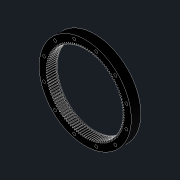
# Autodesk Inventor part: unit-ring_gear
Saved by Autodesk Inventor 2022 (Build 260153000, 153)
## iProperties
Created: 2021-07-12
Part Number: unit-ring_gear
Material: ABS プラスチック
Document SubType Name: Modeling
Designer: yuta0
Density: 1.06 g/cm^3
Appearance: 滑らか - 黒
Mass: 40.8022 g
Surface Area: 244.347 cm^2
Volume: 38.4926 cm^3
購入先: 印刷
在庫数: 0.0
Author: yuta0
Autodesk Inventor part; units mm, degrees
ref_plane "YZ Plane" through (0, 0, 0) normal (1, 0, 0) x (0, 1, 0)
ref_plane "XZ Plane" through (0, 0, 0) normal (0, 1, 0) x (-1, 0, 0)
ref_plane "XY Plane" through (0, 0, 0) normal (0, 0, 1) x (1, 0, 0)
sketch "スケッチ1" plane through (0, 0, 0) normal (0, 0, 1) x (1, 0, 0)
  circle A0 centre (0, 0) radius 67.5
  arc A1 (3.6193, -57.2712) -> (4.2488, -54.9715) centre (-9.8202, -52.3566) ccw
  arc A2 (2.8158, -57.3163) -> (3.6193, -57.2712) centre (0, 0) ccw
  arc A3 (1.9328, -55.1015) -> (2.8158, -57.3163) centre (15.6206, -50.9279) ccw
  arc A4 (1.1598, -55.1232) -> (1.9328, -55.1015) centre (0, 0) ccw
  arc A5 (0.4024, -57.384) -> (1.1598, -55.1232) centre (-12.7405, -51.7236) ccw
  arc A6 (-0.4024, -57.384) -> (0.4024, -57.384) centre (0, 0) ccw
  arc A7 (-1.1598, -55.1232) -> (-0.4024, -57.384) centre (12.7405, -51.7236) ccw
  arc A8 (-1.9328, -55.1015) -> (-1.1598, -55.1232) centre (0, 0) ccw
  arc A9 (-2.8158, -57.3163) -> (-1.9328, -55.1015) centre (-15.6206, -50.9279) ccw
  arc A10 (-3.6193, -57.2712) -> (-2.8158, -57.3163) centre (0, 0) ccw
  arc A11 (-4.2488, -54.9715) -> (-3.6193, -57.2712) centre (9.8202, -52.3566) ccw
  arc A12 (-5.0193, -54.9065) -> (-4.2488, -54.9715) centre (0, 0) ccw
  arc A13 (-6.0251, -57.0682) -> (-5.0193, -54.9065) centre (-18.4516, -49.9719) ccw
  arc A14 (-6.8249, -56.9781) -> (-6.0251, -57.0682) centre (0, 0) ccw
  arc A15 (-7.3244, -54.6468) -> (-6.8249, -56.9781) centre (6.8691, -52.8248) ccw
  arc A16 (-8.09, -54.5387) -> (-7.3244, -54.6468) centre (0, 0) ccw
  arc A17 (-9.2155, -56.6406) -> (-8.09, -54.5387) centre (-21.2245, -48.8587) ccw
  arc A18 (-10.0089, -56.5058) -> (-9.2155, -56.6406) centre (0, 0) ccw
  arc A19 (-10.3769, -54.1501) -> (-10.0089, -56.5058) centre (3.8964, -53.1269) ccw
  arc A20 (-11.1353, -53.9992) -> (-10.3769, -54.1501) centre (0, 0) ccw
  arc A21 (-12.3768, -56.0348) -> (-11.1353, -53.9992) centre (-23.9306, -47.5918) ccw
  arc A22 (-13.1615, -55.8557) -> (-12.3768, -56.0348) centre (0, 0) ccw
  arc A23 (-13.3968, -53.4831) -> (-13.1615, -55.8557) centre (0.9114, -53.2618) ccw
  arc A24 (-14.1456, -53.2899) -> (-13.3968, -53.4831) centre (0, 0) ccw
  arc A25 (-15.4992, -55.2527) -> (-14.1456, -53.2899) centre (-26.5615, -46.1751) ccw
  arc A26 (-16.2726, -55.0299) -> (-15.4992, -55.2527) centre (0, 0) ccw
  arc A27 (-16.3746, -52.6478) -> (-16.2726, -55.0299) centre (-2.0764, -53.2291) ccw
  arc A28 (-17.1113, -52.4129) -> (-16.3746, -52.6478) centre (0, 0) ccw
  arc A29 (-18.5729, -54.2967) -> (-17.1113, -52.4129) centre (-29.1087, -44.6131) ccw
  arc A30 (-19.3326, -54.0309) -> (-18.5729, -54.2967) centre (0, 0) ccw
  arc A31 (-19.3008, -51.6468) -> (-19.3326, -54.0309) centre (-5.0577, -53.0289) ccw
  arc A32 (-20.0232, -51.3711) -> (-19.3008, -51.6468) centre (0, 0) ccw
  arc A33 (-21.5881, -53.1699) -> (-20.0232, -51.3711) centre (-31.5644, -42.9108) ccw
  arc A34 (-22.3317, -52.8619) -> (-21.5881, -53.1699) centre (0, 0) ccw
  arc A35 (-22.1663, -50.4834) -> (-22.3317, -52.8619) centre (-8.0231, -52.6619) ccw
  arc A36 (-22.8721, -50.1675) -> (-22.1663, -50.4834) centre (0, 0) ccw
  arc A37 (-24.5354, -51.8758) -> (-22.8721, -50.1675) centre (-33.9208, -41.0735) ccw
  arc A38 (-25.2605, -51.5266) -> (-24.5354, -51.8758) centre (0, 0) ccw
  arc A39 (-24.962, -49.1611) -> (-25.2605, -51.5266) centre (-10.9633, -52.1292) ccw
  arc A40 (-25.649, -48.8062) -> (-24.962, -49.1611) centre (0, 0) ccw
  arc A41 (-27.4055, -50.4185) -> (-25.649, -48.8062) centre (-36.1704, -39.1069) ccw
  arc A42 (-28.1099, -50.0292) -> (-27.4055, -50.4185) centre (0, 0) ccw
  arc A43 (-27.6792, -47.6841) -> (-28.1099, -50.0292) centre (-13.8689, -51.4325) ccw
  arc A44 (-28.3453, -47.2912) -> (-27.6792, -47.6841) centre (0, 0) ccw
  arc A45 (-30.1894, -48.8025) -> (-28.3453, -47.2912) centre (-38.3063, -37.0173) ccw
  arc A46 (-30.8709, -48.3743) -> (-30.1894, -48.8025) centre (0, 0) ccw
  arc A47 (-30.3094, -46.0571) -> (-30.8709, -48.3743) centre (-16.731, -50.574) ccw
  arc A48 (-30.9523, -45.6275) -> (-30.3094, -46.0571) centre (0, 0) ccw
  arc A49 (-32.8783, -47.033) -> (-30.9523, -45.6275) centre (-40.3216, -34.8112) ccw
  arc A50 (-33.5347, -46.5673) -> (-32.8783, -47.033) centre (0, 0) ccw
  arc A51 (-32.8441, -44.2852) -> (-33.5347, -46.5673) centre (-19.5403, -49.5563) ccw
  arc A52 (-33.462, -43.8202) -> (-32.8441, -44.2852) centre (0, 0) ccw
  arc A53 (-35.4637, -45.1155) -> (-33.462, -43.8202) centre (-42.21, -32.4956) ccw
  arc A54 (-36.093, -44.6137) -> (-35.4637, -45.1155) centre (0, 0) ccw
  arc A55 (-35.2755, -42.3739) -> (-36.093, -44.6137) centre (-22.2882, -48.3827) ccw
  arc A56 (-35.8664, -41.875) -> (-35.2755, -42.3739) centre (0, 0) ccw
  arc A57 (-37.9376, -43.0561) -> (-35.8664, -41.875) centre (-43.9657, -30.0777) ccw
  arc A58 (-38.5377, -42.5198) -> (-37.9376, -43.0561) centre (0, 0) ccw
  arc A59 (-37.596, -40.3293) -> (-38.5377, -42.5198) centre (-24.966, -47.0569) ccw
  arc A60 (-38.1579, -39.7981) -> (-37.596, -40.3293) centre (0, 0) ccw
  arc A61 (-40.2921, -40.8612) -> (-38.1579, -39.7981) centre (-45.583, -27.5652) ccw
  arc A62 (-40.8612, -40.2921) -> (-40.2921, -40.8612) centre (0, 0) ccw
  arc A63 (-39.7981, -38.1579) -> (-40.8612, -40.2921) centre (-27.5652, -45.583) ccw
  arc A64 (-40.3293, -37.596) -> (-39.7981, -38.1579) centre (0, 0) ccw
  arc A65 (-42.5198, -38.5377) -> (-40.3293, -37.596) centre (-47.0569, -24.966) ccw
  arc A66 (-43.0561, -37.9376) -> (-42.5198, -38.5377) centre (0, 0) ccw
  arc A67 (-41.875, -35.8664) -> (-43.0561, -37.9376) centre (-30.0777, -43.9657) ccw
  arc A68 (-42.3739, -35.2755) -> (-41.875, -35.8664) centre (0, 0) ccw
  arc A69 (-44.6137, -36.093) -> (-42.3739, -35.2755) centre (-48.3827, -22.2882) ccw
  arc A70 (-45.1155, -35.4637) -> (-44.6137, -36.093) centre (0, 0) ccw
  arc A71 (-43.8202, -33.462) -> (-45.1155, -35.4637) centre (-32.4956, -42.21) ccw
  arc A72 (-44.2852, -32.8441) -> (-43.8202, -33.462) centre (0, 0) ccw
  arc A73 (-46.5673, -33.5347) -> (-44.2852, -32.8441) centre (-49.5563, -19.5403) ccw
  arc A74 (-47.033, -32.8783) -> (-46.5673, -33.5347) centre (0, 0) ccw
  arc A75 (-45.6275, -30.9523) -> (-47.033, -32.8783) centre (-34.8112, -40.3216) ccw
  arc A76 (-46.0571, -30.3094) -> (-45.6275, -30.9523) centre (0, 0) ccw
  arc A77 (-48.3743, -30.8709) -> (-46.0571, -30.3094) centre (-50.574, -16.731) ccw
  arc A78 (-48.8025, -30.1894) -> (-48.3743, -30.8709) centre (0, 0) ccw
  arc A79 (-47.2912, -28.3453) -> (-48.8025, -30.1894) centre (-37.0173, -38.3063) ccw
  arc A80 (-47.6841, -27.6792) -> (-47.2912, -28.3453) centre (0, 0) ccw
  arc A81 (-50.0292, -28.1099) -> (-47.6841, -27.6792) centre (-51.4325, -13.8689) ccw
  arc A82 (-50.4185, -27.4055) -> (-50.0292, -28.1099) centre (0, 0) ccw
  arc A83 (-48.8062, -25.649) -> (-50.4185, -27.4055) centre (-39.1069, -36.1704) ccw
  arc A84 (-49.1611, -24.962) -> (-48.8062, -25.649) centre (0, 0) ccw
  arc A85 (-51.5266, -25.2605) -> (-49.1611, -24.962) centre (-52.1292, -10.9633) ccw
  arc A86 (-51.8758, -24.5354) -> (-51.5266, -25.2605) centre (0, 0) ccw
  arc A87 (-50.1675, -22.8721) -> (-51.8758, -24.5354) centre (-41.0735, -33.9208) ccw
  arc A88 (-50.4834, -22.1663) -> (-50.1675, -22.8721) centre (0, 0) ccw
  arc A89 (-52.8619, -22.3317) -> (-50.4834, -22.1663) centre (-52.6619, -8.0231) ccw
  arc A90 (-53.1699, -21.5881) -> (-52.8619, -22.3317) centre (0, 0) ccw
  arc A91 (-51.3711, -20.0232) -> (-53.1699, -21.5881) centre (-42.9108, -31.5644) ccw
  arc A92 (-51.6468, -19.3008) -> (-51.3711, -20.0232) centre (0, 0) ccw
  arc A93 (-54.0309, -19.3326) -> (-51.6468, -19.3008) centre (-53.0289, -5.0577) ccw
  arc A94 (-54.2967, -18.5729) -> (-54.0309, -19.3326) centre (0, 0) ccw
  arc A95 (-52.4129, -17.1113) -> (-54.2967, -18.5729) centre (-44.6131, -29.1087) ccw
  arc A96 (-52.6478, -16.3746) -> (-52.4129, -17.1113) centre (0, 0) ccw
  arc A97 (-55.0299, -16.2726) -> (-52.6478, -16.3746) centre (-53.2291, -2.0764) ccw
  arc A98 (-55.2527, -15.4992) -> (-55.0299, -16.2726) centre (0, 0) ccw
  arc A99 (-53.2899, -14.1456) -> (-55.2527, -15.4992) centre (-46.1751, -26.5615) ccw
  arc A100 (-53.4831, -13.3968) -> (-53.2899, -14.1456) centre (0, 0) ccw
  arc A101 (-55.8557, -13.1615) -> (-53.4831, -13.3968) centre (-53.2618, 0.9114) ccw
  arc A102 (-56.0348, -12.3768) -> (-55.8557, -13.1615) centre (0, 0) ccw
  arc A103 (-53.9992, -11.1353) -> (-56.0348, -12.3768) centre (-47.5918, -23.9306) ccw
  arc A104 (-54.1501, -10.3769) -> (-53.9992, -11.1353) centre (0, 0) ccw
  arc A105 (-56.5058, -10.0089) -> (-54.1501, -10.3769) centre (-53.1269, 3.8964) ccw
  arc A106 (-56.6406, -9.2155) -> (-56.5058, -10.0089) centre (0, 0) ccw
  arc A107 (-54.5387, -8.09) -> (-56.6406, -9.2155) centre (-48.8587, -21.2245) ccw
  arc A108 (-54.6468, -7.3244) -> (-54.5387, -8.09) centre (0, 0) ccw
  arc A109 (-56.9781, -6.8249) -> (-54.6468, -7.3244) centre (-52.8248, 6.8691) ccw
  arc A110 (-57.0682, -6.0251) -> (-56.9781, -6.8249) centre (0, 0) ccw
  arc A111 (-54.9065, -5.0193) -> (-57.0682, -6.0251) centre (-49.9719, -18.4516) ccw
  arc A112 (-54.9715, -4.2488) -> (-54.9065, -5.0193) centre (0, 0) ccw
  arc A113 (-57.2712, -3.6193) -> (-54.9715, -4.2488) centre (-52.3566, 9.8202) ccw
  arc A114 (-57.3163, -2.8158) -> (-57.2712, -3.6193) centre (0, 0) ccw
  arc A115 (-55.1015, -1.9328) -> (-57.3163, -2.8158) centre (-50.9279, -15.6206) ccw
  arc A116 (-55.1232, -1.1598) -> (-55.1015, -1.9328) centre (0, 0) ccw
  arc A117 (-57.384, -0.4024) -> (-55.1232, -1.1598) centre (-51.7236, 12.7405) ccw
  arc A118 (-57.384, 0.4024) -> (-57.384, -0.4024) centre (0, 0) ccw
  arc A119 (-55.1232, 1.1598) -> (-57.384, 0.4024) centre (-51.7236, -12.7405) ccw
  arc A120 (-55.1015, 1.9328) -> (-55.1232, 1.1598) centre (0, 0) ccw
  arc A121 (-57.3163, 2.8158) -> (-55.1015, 1.9328) centre (-50.9279, 15.6206) ccw
  arc A122 (-57.2712, 3.6193) -> (-57.3163, 2.8158) centre (0, 0) ccw
  arc A123 (-54.9715, 4.2488) -> (-57.2712, 3.6193) centre (-52.3566, -9.8202) ccw
  arc A124 (-54.9065, 5.0193) -> (-54.9715, 4.2488) centre (0, 0) ccw
  arc A125 (-57.0682, 6.0251) -> (-54.9065, 5.0193) centre (-49.9719, 18.4516) ccw
  arc A126 (-56.9781, 6.8249) -> (-57.0682, 6.0251) centre (0, 0) ccw
  arc A127 (-54.6468, 7.3244) -> (-56.9781, 6.8249) centre (-52.8248, -6.8691) ccw
  arc A128 (-54.5387, 8.09) -> (-54.6468, 7.3244) centre (0, 0) ccw
  arc A129 (-56.6406, 9.2155) -> (-54.5387, 8.09) centre (-48.8587, 21.2245) ccw
  arc A130 (-56.5058, 10.0089) -> (-56.6406, 9.2155) centre (0, 0) ccw
  arc A131 (-54.1501, 10.3769) -> (-56.5058, 10.0089) centre (-53.1269, -3.8964) ccw
  arc A132 (-53.9992, 11.1353) -> (-54.1501, 10.3769) centre (0, 0) ccw
  arc A133 (-56.0348, 12.3768) -> (-53.9992, 11.1353) centre (-47.5918, 23.9306) ccw
  arc A134 (-55.8557, 13.1615) -> (-56.0348, 12.3768) centre (0, 0) ccw
  arc A135 (-53.4831, 13.3968) -> (-55.8557, 13.1615) centre (-53.2618, -0.9114) ccw
  arc A136 (-53.2899, 14.1456) -> (-53.4831, 13.3968) centre (0, 0) ccw
  arc A137 (-55.2527, 15.4992) -> (-53.2899, 14.1456) centre (-46.1751, 26.5615) ccw
  arc A138 (-55.0299, 16.2726) -> (-55.2527, 15.4992) centre (0, 0) ccw
  arc A139 (-52.6478, 16.3746) -> (-55.0299, 16.2726) centre (-53.2291, 2.0764) ccw
  arc A140 (-52.4129, 17.1113) -> (-52.6478, 16.3746) centre (0, 0) ccw
  arc A141 (-54.2967, 18.5729) -> (-52.4129, 17.1113) centre (-44.6131, 29.1087) ccw
  arc A142 (-54.0309, 19.3326) -> (-54.2967, 18.5729) centre (0, 0) ccw
  arc A143 (-51.6468, 19.3008) -> (-54.0309, 19.3326) centre (-53.0289, 5.0577) ccw
  arc A144 (-51.3711, 20.0232) -> (-51.6468, 19.3008) centre (0, 0) ccw
  arc A145 (-53.1699, 21.5881) -> (-51.3711, 20.0232) centre (-42.9108, 31.5644) ccw
  arc A146 (-52.8619, 22.3317) -> (-53.1699, 21.5881) centre (0, 0) ccw
  arc A147 (-50.4834, 22.1663) -> (-52.8619, 22.3317) centre (-52.6619, 8.0231) ccw
  arc A148 (-50.1675, 22.8721) -> (-50.4834, 22.1663) centre (0, 0) ccw
  arc A149 (-51.8758, 24.5354) -> (-50.1675, 22.8721) centre (-41.0735, 33.9208) ccw
  arc A150 (-51.5266, 25.2605) -> (-51.8758, 24.5354) centre (0, 0) ccw
  arc A151 (-49.1611, 24.962) -> (-51.5266, 25.2605) centre (-52.1292, 10.9633) ccw
  arc A152 (-48.8062, 25.649) -> (-49.1611, 24.962) centre (0, 0) ccw
  arc A153 (-50.4185, 27.4055) -> (-48.8062, 25.649) centre (-39.1069, 36.1704) ccw
  arc A154 (-50.0292, 28.1099) -> (-50.4185, 27.4055) centre (0, 0) ccw
  arc A155 (-47.6841, 27.6792) -> (-50.0292, 28.1099) centre (-51.4325, 13.8689) ccw
  arc A156 (-47.2912, 28.3453) -> (-47.6841, 27.6792) centre (0, 0) ccw
  arc A157 (-48.8025, 30.1894) -> (-47.2912, 28.3453) centre (-37.0173, 38.3063) ccw
  arc A158 (-48.3743, 30.8709) -> (-48.8025, 30.1894) centre (0, 0) ccw
  arc A159 (-46.0571, 30.3094) -> (-48.3743, 30.8709) centre (-50.574, 16.731) ccw
  arc A160 (-45.6275, 30.9523) -> (-46.0571, 30.3094) centre (0, 0) ccw
  arc A161 (-47.033, 32.8783) -> (-45.6275, 30.9523) centre (-34.8112, 40.3216) ccw
  arc A162 (-46.5673, 33.5347) -> (-47.033, 32.8783) centre (0, 0) ccw
  arc A163 (-44.2852, 32.8441) -> (-46.5673, 33.5347) centre (-49.5563, 19.5403) ccw
  arc A164 (-43.8202, 33.462) -> (-44.2852, 32.8441) centre (0, 0) ccw
  arc A165 (-45.1155, 35.4637) -> (-43.8202, 33.462) centre (-32.4956, 42.21) ccw
  arc A166 (-44.6137, 36.093) -> (-45.1155, 35.4637) centre (0, 0) ccw
  arc A167 (-42.3739, 35.2755) -> (-44.6137, 36.093) centre (-48.3827, 22.2882) ccw
  arc A168 (-41.875, 35.8664) -> (-42.3739, 35.2755) centre (0, 0) ccw
  arc A169 (-43.0561, 37.9376) -> (-41.875, 35.8664) centre (-30.0777, 43.9657) ccw
  arc A170 (-42.5198, 38.5377) -> (-43.0561, 37.9376) centre (0, 0) ccw
  arc A171 (-40.3293, 37.596) -> (-42.5198, 38.5377) centre (-47.0569, 24.966) ccw
  arc A172 (-39.7981, 38.1579) -> (-40.3293, 37.596) centre (0, 0) ccw
  arc A173 (-40.8612, 40.2921) -> (-39.7981, 38.1579) centre (-27.5652, 45.583) ccw
  arc A174 (-40.2921, 40.8612) -> (-40.8612, 40.2921) centre (0, 0) ccw
  arc A175 (-38.1579, 39.7981) -> (-40.2921, 40.8612) centre (-45.583, 27.5652) ccw
  arc A176 (-37.596, 40.3293) -> (-38.1579, 39.7981) centre (0, 0) ccw
  arc A177 (-38.5377, 42.5198) -> (-37.596, 40.3293) centre (-24.966, 47.0569) ccw
  arc A178 (-37.9376, 43.0561) -> (-38.5377, 42.5198) centre (0, 0) ccw
  arc A179 (-35.8664, 41.875) -> (-37.9376, 43.0561) centre (-43.9657, 30.0777) ccw
  arc A180 (-35.2755, 42.3739) -> (-35.8664, 41.875) centre (0, 0) ccw
  arc A181 (-36.093, 44.6137) -> (-35.2755, 42.3739) centre (-22.2882, 48.3827) ccw
  arc A182 (-35.4637, 45.1155) -> (-36.093, 44.6137) centre (0, 0) ccw
  arc A183 (-33.462, 43.8202) -> (-35.4637, 45.1155) centre (-42.21, 32.4956) ccw
  arc A184 (-32.8441, 44.2852) -> (-33.462, 43.8202) centre (0, 0) ccw
  arc A185 (-33.5347, 46.5673) -> (-32.8441, 44.2852) centre (-19.5403, 49.5563) ccw
  arc A186 (-32.8783, 47.033) -> (-33.5347, 46.5673) centre (0, 0) ccw
  arc A187 (-30.9523, 45.6275) -> (-32.8783, 47.033) centre (-40.3216, 34.8112) ccw
  arc A188 (-30.3094, 46.0571) -> (-30.9523, 45.6275) centre (0, 0) ccw
  arc A189 (-30.8709, 48.3743) -> (-30.3094, 46.0571) centre (-16.731, 50.574) ccw
  arc A190 (-30.1894, 48.8025) -> (-30.8709, 48.3743) centre (0, 0) ccw
  arc A191 (-28.3453, 47.2912) -> (-30.1894, 48.8025) centre (-38.3063, 37.0173) ccw
  arc A192 (-27.6792, 47.6841) -> (-28.3453, 47.2912) centre (0, 0) ccw
  arc A193 (-28.1099, 50.0292) -> (-27.6792, 47.6841) centre (-13.8689, 51.4325) ccw
  arc A194 (-27.4055, 50.4185) -> (-28.1099, 50.0292) centre (0, 0) ccw
  arc A195 (-25.649, 48.8062) -> (-27.4055, 50.4185) centre (-36.1704, 39.1069) ccw
  arc A196 (-24.962, 49.1611) -> (-25.649, 48.8062) centre (0, 0) ccw
  arc A197 (-25.2605, 51.5266) -> (-24.962, 49.1611) centre (-10.9633, 52.1292) ccw
  arc A198 (-24.5354, 51.8758) -> (-25.2605, 51.5266) centre (0, 0) ccw
  arc A199 (-22.8721, 50.1675) -> (-24.5354, 51.8758) centre (-33.9208, 41.0735) ccw
  arc A200 (-22.1663, 50.4834) -> (-22.8721, 50.1675) centre (0, 0) ccw
  arc A201 (-22.3317, 52.8619) -> (-22.1663, 50.4834) centre (-8.0231, 52.6619) ccw
  arc A202 (-21.5881, 53.1699) -> (-22.3317, 52.8619) centre (0, 0) ccw
  arc A203 (-20.0232, 51.3711) -> (-21.5881, 53.1699) centre (-31.5644, 42.9108) ccw
  arc A204 (-19.3008, 51.6468) -> (-20.0232, 51.3711) centre (0, 0) ccw
  arc A205 (-19.3326, 54.0309) -> (-19.3008, 51.6468) centre (-5.0577, 53.0289) ccw
  arc A206 (-18.5729, 54.2967) -> (-19.3326, 54.0309) centre (0, 0) ccw
  arc A207 (-17.1113, 52.4129) -> (-18.5729, 54.2967) centre (-29.1087, 44.6131) ccw
  arc A208 (-16.3746, 52.6478) -> (-17.1113, 52.4129) centre (0, 0) ccw
  arc A209 (-16.2726, 55.0299) -> (-16.3746, 52.6478) centre (-2.0764, 53.2291) ccw
  arc A210 (-15.4992, 55.2527) -> (-16.2726, 55.0299) centre (0, 0) ccw
  arc A211 (-14.1456, 53.2899) -> (-15.4992, 55.2527) centre (-26.5615, 46.1751) ccw
  arc A212 (-13.3968, 53.4831) -> (-14.1456, 53.2899) centre (0, 0) ccw
  arc A213 (-13.1615, 55.8557) -> (-13.3968, 53.4831) centre (0.9114, 53.2618) ccw
  arc A214 (-12.3768, 56.0348) -> (-13.1615, 55.8557) centre (0, 0) ccw
  arc A215 (-11.1353, 53.9992) -> (-12.3768, 56.0348) centre (-23.9306, 47.5918) ccw
  arc A216 (-10.3769, 54.1501) -> (-11.1353, 53.9992) centre (0, 0) ccw
  arc A217 (-10.0089, 56.5058) -> (-10.3769, 54.1501) centre (3.8964, 53.1269) ccw
  arc A218 (-9.2155, 56.6406) -> (-10.0089, 56.5058) centre (0, 0) ccw
  arc A219 (-8.09, 54.5387) -> (-9.2155, 56.6406) centre (-21.2245, 48.8587) ccw
  arc A220 (-7.3244, 54.6468) -> (-8.09, 54.5387) centre (0, 0) ccw
  arc A221 (-6.8249, 56.9781) -> (-7.3244, 54.6468) centre (6.8691, 52.8248) ccw
  arc A222 (-6.0251, 57.0682) -> (-6.8249, 56.9781) centre (0, 0) ccw
  arc A223 (-5.0193, 54.9065) -> (-6.0251, 57.0682) centre (-18.4516, 49.9719) ccw
  arc A224 (-4.2488, 54.9715) -> (-5.0193, 54.9065) centre (0, 0) ccw
  arc A225 (-3.6193, 57.2712) -> (-4.2488, 54.9715) centre (9.8202, 52.3566) ccw
  arc A226 (-2.8158, 57.3163) -> (-3.6193, 57.2712) centre (0, 0) ccw
  arc A227 (-1.9328, 55.1015) -> (-2.8158, 57.3163) centre (-15.6206, 50.9279) ccw
  arc A228 (-1.1598, 55.1232) -> (-1.9328, 55.1015) centre (0, 0) ccw
  arc A229 (-0.4024, 57.384) -> (-1.1598, 55.1232) centre (12.7405, 51.7236) ccw
  arc A230 (0.4024, 57.384) -> (-0.4024, 57.384) centre (0, 0) ccw
  arc A231 (1.1598, 55.1232) -> (0.4024, 57.384) centre (-12.7405, 51.7236) ccw
  arc A232 (1.9328, 55.1015) -> (1.1598, 55.1232) centre (0, 0) ccw
  arc A233 (2.8158, 57.3163) -> (1.9328, 55.1015) centre (15.6206, 50.9279) ccw
  arc A234 (3.6193, 57.2712) -> (2.8158, 57.3163) centre (0, 0) ccw
  arc A235 (4.2488, 54.9715) -> (3.6193, 57.2712) centre (-9.8202, 52.3566) ccw
  arc A236 (5.0193, 54.9065) -> (4.2488, 54.9715) centre (0, 0) ccw
  arc A237 (6.0251, 57.0682) -> (5.0193, 54.9065) centre (18.4516, 49.9719) ccw
  arc A238 (6.8249, 56.9781) -> (6.0251, 57.0682) centre (0, 0) ccw
  arc A239 (7.3244, 54.6468) -> (6.8249, 56.9781) centre (-6.8691, 52.8248) ccw
  arc A240 (8.09, 54.5387) -> (7.3244, 54.6468) centre (0, 0) ccw
  arc A241 (9.2155, 56.6406) -> (8.09, 54.5387) centre (21.2245, 48.8587) ccw
  arc A242 (10.0089, 56.5058) -> (9.2155, 56.6406) centre (0, 0) ccw
  arc A243 (10.3769, 54.1501) -> (10.0089, 56.5058) centre (-3.8964, 53.1269) ccw
  arc A244 (11.1353, 53.9992) -> (10.3769, 54.1501) centre (0, 0) ccw
  arc A245 (12.3768, 56.0348) -> (11.1353, 53.9992) centre (23.9306, 47.5918) ccw
  arc A246 (13.1615, 55.8557) -> (12.3768, 56.0348) centre (0, 0) ccw
  arc A247 (13.3968, 53.4831) -> (13.1615, 55.8557) centre (-0.9114, 53.2618) ccw
  arc A248 (14.1456, 53.2899) -> (13.3968, 53.4831) centre (0, 0) ccw
  arc A249 (15.4992, 55.2527) -> (14.1456, 53.2899) centre (26.5615, 46.1751) ccw
  arc A250 (16.2726, 55.0299) -> (15.4992, 55.2527) centre (0, 0) ccw
  arc A251 (16.3746, 52.6478) -> (16.2726, 55.0299) centre (2.0764, 53.2291) ccw
  arc A252 (17.1113, 52.4129) -> (16.3746, 52.6478) centre (0, 0) ccw
  arc A253 (18.5729, 54.2967) -> (17.1113, 52.4129) centre (29.1087, 44.6131) ccw
  arc A254 (19.3326, 54.0309) -> (18.5729, 54.2967) centre (0, 0) ccw
  arc A255 (19.3008, 51.6468) -> (19.3326, 54.0309) centre (5.0577, 53.0289) ccw
  arc A256 (20.0232, 51.3711) -> (19.3008, 51.6468) centre (0, 0) ccw
  arc A257 (21.5881, 53.1699) -> (20.0232, 51.3711) centre (31.5644, 42.9108) ccw
  arc A258 (22.3317, 52.8619) -> (21.5881, 53.1699) centre (0, 0) ccw
  arc A259 (22.1663, 50.4834) -> (22.3317, 52.8619) centre (8.0231, 52.6619) ccw
  arc A260 (22.8721, 50.1675) -> (22.1663, 50.4834) centre (0, 0) ccw
  arc A261 (24.5354, 51.8758) -> (22.8721, 50.1675) centre (33.9208, 41.0735) ccw
  arc A262 (25.2605, 51.5266) -> (24.5354, 51.8758) centre (0, 0) ccw
  arc A263 (24.962, 49.1611) -> (25.2605, 51.5266) centre (10.9633, 52.1292) ccw
  arc A264 (25.649, 48.8062) -> (24.962, 49.1611) centre (0, 0) ccw
  arc A265 (27.4055, 50.4185) -> (25.649, 48.8062) centre (36.1704, 39.1069) ccw
  arc A266 (28.1099, 50.0292) -> (27.4055, 50.4185) centre (0, 0) ccw
  arc A267 (27.6792, 47.6841) -> (28.1099, 50.0292) centre (13.8689, 51.4325) ccw
  arc A268 (28.3453, 47.2912) -> (27.6792, 47.6841) centre (0, 0) ccw
  arc A269 (30.1894, 48.8025) -> (28.3453, 47.2912) centre (38.3063, 37.0173) ccw
  arc A270 (30.8709, 48.3743) -> (30.1894, 48.8025) centre (0, 0) ccw
  arc A271 (30.3094, 46.0571) -> (30.8709, 48.3743) centre (16.731, 50.574) ccw
  arc A272 (30.9523, 45.6275) -> (30.3094, 46.0571) centre (0, 0) ccw
  arc A273 (32.8783, 47.033) -> (30.9523, 45.6275) centre (40.3216, 34.8112) ccw
  arc A274 (33.5347, 46.5673) -> (32.8783, 47.033) centre (0, 0) ccw
  arc A275 (32.8441, 44.2852) -> (33.5347, 46.5673) centre (19.5403, 49.5563) ccw
  arc A276 (33.462, 43.8202) -> (32.8441, 44.2852) centre (0, 0) ccw
  arc A277 (35.4637, 45.1155) -> (33.462, 43.8202) centre (42.21, 32.4956) ccw
  arc A278 (36.093, 44.6137) -> (35.4637, 45.1155) centre (0, 0) ccw
  arc A279 (35.2755, 42.3739) -> (36.093, 44.6137) centre (22.2882, 48.3827) ccw
  arc A280 (35.8664, 41.875) -> (35.2755, 42.3739) centre (0, 0) ccw
  arc A281 (37.9376, 43.0561) -> (35.8664, 41.875) centre (43.9657, 30.0777) ccw
  arc A282 (38.5377, 42.5198) -> (37.9376, 43.0561) centre (0, 0) ccw
  arc A283 (37.596, 40.3293) -> (38.5377, 42.5198) centre (24.966, 47.0569) ccw
  arc A284 (38.1579, 39.7981) -> (37.596, 40.3293) centre (0, 0) ccw
  arc A285 (40.2921, 40.8612) -> (38.1579, 39.7981) centre (45.583, 27.5652) ccw
  arc A286 (40.8612, 40.2921) -> (40.2921, 40.8612) centre (0, 0) ccw
  arc A287 (39.7981, 38.1579) -> (40.8612, 40.2921) centre (27.5652, 45.583) ccw
  arc A288 (40.3293, 37.596) -> (39.7981, 38.1579) centre (0, 0) ccw
  arc A289 (42.5198, 38.5377) -> (40.3293, 37.596) centre (47.0569, 24.966) ccw
  arc A290 (43.0561, 37.9376) -> (42.5198, 38.5377) centre (0, 0) ccw
  arc A291 (41.875, 35.8664) -> (43.0561, 37.9376) centre (30.0777, 43.9657) ccw
  arc A292 (42.3739, 35.2755) -> (41.875, 35.8664) centre (0, 0) ccw
  arc A293 (44.6137, 36.093) -> (42.3739, 35.2755) centre (48.3827, 22.2882) ccw
  arc A294 (45.1155, 35.4637) -> (44.6137, 36.093) centre (0, 0) ccw
  arc A295 (43.8202, 33.462) -> (45.1155, 35.4637) centre (32.4956, 42.21) ccw
  arc A296 (44.2852, 32.8441) -> (43.8202, 33.462) centre (0, 0) ccw
  arc A297 (46.5673, 33.5347) -> (44.2852, 32.8441) centre (49.5563, 19.5403) ccw
  arc A298 (47.033, 32.8783) -> (46.5673, 33.5347) centre (0, 0) ccw
  arc A299 (45.6275, 30.9523) -> (47.033, 32.8783) centre (34.8112, 40.3216) ccw
  arc A300 (46.0571, 30.3094) -> (45.6275, 30.9523) centre (0, 0) ccw
  arc A301 (48.3743, 30.8709) -> (46.0571, 30.3094) centre (50.574, 16.731) ccw
  arc A302 (48.8025, 30.1894) -> (48.3743, 30.8709) centre (0, 0) ccw
  arc A303 (47.2912, 28.3453) -> (48.8025, 30.1894) centre (37.0173, 38.3063) ccw
  arc A304 (47.6841, 27.6792) -> (47.2912, 28.3453) centre (0, 0) ccw
  arc A305 (50.0292, 28.1099) -> (47.6841, 27.6792) centre (51.4325, 13.8689) ccw
  arc A306 (50.4185, 27.4055) -> (50.0292, 28.1099) centre (0, 0) ccw
  arc A307 (48.8062, 25.649) -> (50.4185, 27.4055) centre (39.1069, 36.1704) ccw
  arc A308 (49.1611, 24.962) -> (48.8062, 25.649) centre (0, 0) ccw
  arc A309 (51.5266, 25.2605) -> (49.1611, 24.962) centre (52.1292, 10.9633) ccw
  arc A310 (51.8758, 24.5354) -> (51.5266, 25.2605) centre (0, 0) ccw
  arc A311 (50.1675, 22.8721) -> (51.8758, 24.5354) centre (41.0735, 33.9208) ccw
  arc A312 (50.4834, 22.1663) -> (50.1675, 22.8721) centre (0, 0) ccw
  arc A313 (52.8619, 22.3317) -> (50.4834, 22.1663) centre (52.6619, 8.0231) ccw
  arc A314 (53.1699, 21.5881) -> (52.8619, 22.3317) centre (0, 0) ccw
  arc A315 (51.3711, 20.0232) -> (53.1699, 21.5881) centre (42.9108, 31.5644) ccw
  arc A316 (51.6468, 19.3008) -> (51.3711, 20.0232) centre (0, 0) ccw
  arc A317 (54.0309, 19.3326) -> (51.6468, 19.3008) centre (53.0289, 5.0577) ccw
  arc A318 (54.2967, 18.5729) -> (54.0309, 19.3326) centre (0, 0) ccw
  arc A319 (52.4129, 17.1113) -> (54.2967, 18.5729) centre (44.6131, 29.1087) ccw
  arc A320 (52.6478, 16.3746) -> (52.4129, 17.1113) centre (0, 0) ccw
  arc A321 (55.0299, 16.2726) -> (52.6478, 16.3746) centre (53.2291, 2.0764) ccw
  arc A322 (55.2527, 15.4992) -> (55.0299, 16.2726) centre (0, 0) ccw
  arc A323 (53.2899, 14.1456) -> (55.2527, 15.4992) centre (46.1751, 26.5615) ccw
  arc A324 (53.4831, 13.3968) -> (53.2899, 14.1456) centre (0, 0) ccw
  arc A325 (55.8557, 13.1615) -> (53.4831, 13.3968) centre (53.2618, -0.9114) ccw
  arc A326 (56.0348, 12.3768) -> (55.8557, 13.1615) centre (0, 0) ccw
  arc A327 (53.9992, 11.1353) -> (56.0348, 12.3768) centre (47.5918, 23.9306) ccw
  arc A328 (54.1501, 10.3769) -> (53.9992, 11.1353) centre (0, 0) ccw
  arc A329 (56.5058, 10.0089) -> (54.1501, 10.3769) centre (53.1269, -3.8964) ccw
  arc A330 (56.6406, 9.2155) -> (56.5058, 10.0089) centre (0, 0) ccw
  arc A331 (54.5387, 8.09) -> (56.6406, 9.2155) centre (48.8587, 21.2245) ccw
  arc A332 (54.6468, 7.3244) -> (54.5387, 8.09) centre (0, 0) ccw
  arc A333 (56.9781, 6.8249) -> (54.6468, 7.3244) centre (52.8248, -6.8691) ccw
  arc A334 (57.0682, 6.0251) -> (56.9781, 6.8249) centre (0, 0) ccw
  arc A335 (54.9065, 5.0193) -> (57.0682, 6.0251) centre (49.9719, 18.4516) ccw
  arc A336 (54.9715, 4.2488) -> (54.9065, 5.0193) centre (0, 0) ccw
  arc A337 (57.2712, 3.6193) -> (54.9715, 4.2488) centre (52.3566, -9.8202) ccw
  arc A338 (57.3163, 2.8158) -> (57.2712, 3.6193) centre (0, 0) ccw
  arc A339 (55.1015, 1.9328) -> (57.3163, 2.8158) centre (50.9279, 15.6206) ccw
  arc A340 (55.1232, 1.1598) -> (55.1015, 1.9328) centre (0, 0) ccw
  arc A341 (57.384, 0.4024) -> (55.1232, 1.1598) centre (51.7236, -12.7405) ccw
  arc A342 (57.384, -0.4024) -> (57.384, 0.4024) centre (0, 0) ccw
  arc A343 (55.1232, -1.1598) -> (57.384, -0.4024) centre (51.7236, 12.7405) ccw
  arc A344 (55.1015, -1.9328) -> (55.1232, -1.1598) centre (0, 0) ccw
  arc A345 (57.3163, -2.8158) -> (55.1015, -1.9328) centre (50.9279, -15.6206) ccw
  arc A346 (57.2712, -3.6193) -> (57.3163, -2.8158) centre (0, 0) ccw
  arc A347 (54.9715, -4.2488) -> (57.2712, -3.6193) centre (52.3566, 9.8202) ccw
  arc A348 (54.9065, -5.0193) -> (54.9715, -4.2488) centre (0, 0) ccw
  arc A349 (57.0682, -6.0251) -> (54.9065, -5.0193) centre (49.9719, -18.4516) ccw
  arc A350 (56.9781, -6.8249) -> (57.0682, -6.0251) centre (0, 0) ccw
  arc A351 (54.6468, -7.3244) -> (56.9781, -6.8249) centre (52.8248, 6.8691) ccw
  arc A352 (54.5387, -8.09) -> (54.6468, -7.3244) centre (0, 0) ccw
  arc A353 (56.6406, -9.2155) -> (54.5387, -8.09) centre (48.8587, -21.2245) ccw
  arc A354 (56.5058, -10.0089) -> (56.6406, -9.2155) centre (0, 0) ccw
  arc A355 (54.1501, -10.3769) -> (56.5058, -10.0089) centre (53.1269, 3.8964) ccw
  arc A356 (53.9992, -11.1353) -> (54.1501, -10.3769) centre (0, 0) ccw
  arc A357 (56.0348, -12.3768) -> (53.9992, -11.1353) centre (47.5918, -23.9306) ccw
  arc A358 (55.8557, -13.1615) -> (56.0348, -12.3768) centre (0, 0) ccw
  arc A359 (53.4831, -13.3968) -> (55.8557, -13.1615) centre (53.2618, 0.9114) ccw
  arc A360 (53.2899, -14.1456) -> (53.4831, -13.3968) centre (0, 0) ccw
  arc A361 (55.2527, -15.4992) -> (53.2899, -14.1456) centre (46.1751, -26.5615) ccw
  arc A362 (55.0299, -16.2726) -> (55.2527, -15.4992) centre (0, 0) ccw
  arc A363 (52.6478, -16.3746) -> (55.0299, -16.2726) centre (53.2291, -2.0764) ccw
  arc A364 (52.4129, -17.1113) -> (52.6478, -16.3746) centre (0, 0) ccw
  arc A365 (54.2967, -18.5729) -> (52.4129, -17.1113) centre (44.6131, -29.1087) ccw
  arc A366 (54.0309, -19.3326) -> (54.2967, -18.5729) centre (0, 0) ccw
  arc A367 (51.6468, -19.3008) -> (54.0309, -19.3326) centre (53.0289, -5.0577) ccw
  arc A368 (51.3711, -20.0232) -> (51.6468, -19.3008) centre (0, 0) ccw
  arc A369 (53.1699, -21.5881) -> (51.3711, -20.0232) centre (42.9108, -31.5644) ccw
  arc A370 (52.8619, -22.3317) -> (53.1699, -21.5881) centre (0, 0) ccw
  arc A371 (50.4834, -22.1663) -> (52.8619, -22.3317) centre (52.6619, -8.0231) ccw
  arc A372 (50.1675, -22.8721) -> (50.4834, -22.1663) centre (0, 0) ccw
  arc A373 (51.8758, -24.5354) -> (50.1675, -22.8721) centre (41.0735, -33.9208) ccw
  arc A374 (51.5266, -25.2605) -> (51.8758, -24.5354) centre (0, 0) ccw
  arc A375 (49.1611, -24.962) -> (51.5266, -25.2605) centre (52.1292, -10.9633) ccw
  arc A376 (48.8062, -25.649) -> (49.1611, -24.962) centre (0, 0) ccw
  arc A377 (50.4185, -27.4055) -> (48.8062, -25.649) centre (39.1069, -36.1704) ccw
  arc A378 (50.0292, -28.1099) -> (50.4185, -27.4055) centre (0, 0) ccw
  arc A379 (47.6841, -27.6792) -> (50.0292, -28.1099) centre (51.4325, -13.8689) ccw
  arc A380 (47.2912, -28.3453) -> (47.6841, -27.6792) centre (0, 0) ccw
  arc A381 (48.8025, -30.1894) -> (47.2912, -28.3453) centre (37.0173, -38.3063) ccw
  arc A382 (48.3743, -30.8709) -> (48.8025, -30.1894) centre (0, 0) ccw
  arc A383 (46.0571, -30.3094) -> (48.3743, -30.8709) centre (50.574, -16.731) ccw
  arc A384 (45.6275, -30.9523) -> (46.0571, -30.3094) centre (0, 0) ccw
  arc A385 (47.033, -32.8783) -> (45.6275, -30.9523) centre (34.8112, -40.3216) ccw
  arc A386 (46.5673, -33.5347) -> (47.033, -32.8783) centre (0, 0) ccw
  arc A387 (44.2852, -32.8441) -> (46.5673, -33.5347) centre (49.5563, -19.5403) ccw
  arc A388 (43.8202, -33.462) -> (44.2852, -32.8441) centre (0, 0) ccw
  arc A389 (45.1155, -35.4637) -> (43.8202, -33.462) centre (32.4956, -42.21) ccw
  arc A390 (44.6137, -36.093) -> (45.1155, -35.4637) centre (0, 0) ccw
  arc A391 (42.3739, -35.2755) -> (44.6137, -36.093) centre (48.3827, -22.2882) ccw
  arc A392 (41.875, -35.8664) -> (42.3739, -35.2755) centre (0, 0) ccw
  arc A393 (43.0561, -37.9376) -> (41.875, -35.8664) centre (30.0777, -43.9657) ccw
  arc A394 (42.5198, -38.5377) -> (43.0561, -37.9376) centre (0, 0) ccw
  arc A395 (40.3293, -37.596) -> (42.5198, -38.5377) centre (47.0569, -24.966) ccw
  arc A396 (39.7981, -38.1579) -> (40.3293, -37.596) centre (0, 0) ccw
  arc A397 (40.8612, -40.2921) -> (39.7981, -38.1579) centre (27.5652, -45.583) ccw
  arc A398 (40.2921, -40.8612) -> (40.8612, -40.2921) centre (0, 0) ccw
  arc A399 (38.1579, -39.7981) -> (40.2921, -40.8612) centre (45.583, -27.5652) ccw
  arc A400 (37.596, -40.3293) -> (38.1579, -39.7981) centre (0, 0) ccw
  arc A401 (38.5377, -42.5198) -> (37.596, -40.3293) centre (24.966, -47.0569) ccw
  arc A402 (37.9376, -43.0561) -> (38.5377, -42.5198) centre (0, 0) ccw
  arc A403 (35.8664, -41.875) -> (37.9376, -43.0561) centre (43.9657, -30.0777) ccw
  arc A404 (35.2755, -42.3739) -> (35.8664, -41.875) centre (0, 0) ccw
  arc A405 (36.093, -44.6137) -> (35.2755, -42.3739) centre (22.2882, -48.3827) ccw
  arc A406 (35.4637, -45.1155) -> (36.093, -44.6137) centre (0, 0) ccw
  arc A407 (33.462, -43.8202) -> (35.4637, -45.1155) centre (42.21, -32.4956) ccw
  arc A408 (32.8441, -44.2852) -> (33.462, -43.8202) centre (0, 0) ccw
  arc A409 (33.5347, -46.5673) -> (32.8441, -44.2852) centre (19.5403, -49.5563) ccw
  arc A410 (32.8783, -47.033) -> (33.5347, -46.5673) centre (0, 0) ccw
  arc A411 (30.9523, -45.6275) -> (32.8783, -47.033) centre (40.3216, -34.8112) ccw
  arc A412 (30.3094, -46.0571) -> (30.9523, -45.6275) centre (0, 0) ccw
  arc A413 (30.8709, -48.3743) -> (30.3094, -46.0571) centre (16.731, -50.574) ccw
  arc A414 (30.1894, -48.8025) -> (30.8709, -48.3743) centre (0, 0) ccw
  arc A415 (28.3453, -47.2912) -> (30.1894, -48.8025) centre (38.3063, -37.0173) ccw
  arc A416 (27.6792, -47.6841) -> (28.3453, -47.2912) centre (0, 0) ccw
  arc A417 (28.1099, -50.0292) -> (27.6792, -47.6841) centre (13.8689, -51.4325) ccw
  arc A418 (27.4055, -50.4185) -> (28.1099, -50.0292) centre (0, 0) ccw
  arc A419 (25.649, -48.8062) -> (27.4055, -50.4185) centre (36.1704, -39.1069) ccw
  arc A420 (24.962, -49.1611) -> (25.649, -48.8062) centre (0, 0) ccw
  arc A421 (25.2605, -51.5266) -> (24.962, -49.1611) centre (10.9633, -52.1292) ccw
  arc A422 (24.5354, -51.8758) -> (25.2605, -51.5266) centre (0, 0) ccw
  arc A423 (22.8721, -50.1675) -> (24.5354, -51.8758) centre (33.9208, -41.0735) ccw
  arc A424 (22.1663, -50.4834) -> (22.8721, -50.1675) centre (0, 0) ccw
  arc A425 (22.3317, -52.8619) -> (22.1663, -50.4834) centre (8.0231, -52.6619) ccw
  arc A426 (21.5881, -53.1699) -> (22.3317, -52.8619) centre (0, 0) ccw
  arc A427 (20.0232, -51.3711) -> (21.5881, -53.1699) centre (31.5644, -42.9108) ccw
  arc A428 (19.3008, -51.6468) -> (20.0232, -51.3711) centre (0, 0) ccw
  arc A429 (19.3326, -54.0309) -> (19.3008, -51.6468) centre (5.0577, -53.0289) ccw
  arc A430 (18.5729, -54.2967) -> (19.3326, -54.0309) centre (0, 0) ccw
  arc A431 (17.1113, -52.4129) -> (18.5729, -54.2967) centre (29.1087, -44.6131) ccw
  arc A432 (16.3746, -52.6478) -> (17.1113, -52.4129) centre (0, 0) ccw
  arc A433 (16.2726, -55.0299) -> (16.3746, -52.6478) centre (2.0764, -53.2291) ccw
  arc A434 (15.4992, -55.2527) -> (16.2726, -55.0299) centre (0, 0) ccw
  arc A435 (14.1456, -53.2899) -> (15.4992, -55.2527) centre (26.5615, -46.1751) ccw
  arc A436 (13.3968, -53.4831) -> (14.1456, -53.2899) centre (0, 0) ccw
  arc A437 (13.1615, -55.8557) -> (13.3968, -53.4831) centre (-0.9114, -53.2618) ccw
  arc A438 (12.3768, -56.0348) -> (13.1615, -55.8557) centre (0, 0) ccw
  arc A439 (11.1353, -53.9992) -> (12.3768, -56.0348) centre (23.9306, -47.5918) ccw
  arc A440 (10.3769, -54.1501) -> (11.1353, -53.9992) centre (0, 0) ccw
  arc A441 (10.0089, -56.5058) -> (10.3769, -54.1501) centre (-3.8964, -53.1269) ccw
  arc A442 (9.2155, -56.6406) -> (10.0089, -56.5058) centre (0, 0) ccw
  arc A443 (8.09, -54.5387) -> (9.2155, -56.6406) centre (21.2245, -48.8587) ccw
  arc A444 (7.3244, -54.6468) -> (8.09, -54.5387) centre (0, 0) ccw
  arc A445 (6.8249, -56.9781) -> (7.3244, -54.6468) centre (-6.8691, -52.8248) ccw
  arc A446 (6.0251, -57.0682) -> (6.8249, -56.9781) centre (0, 0) ccw
  arc A447 (5.0193, -54.9065) -> (6.0251, -57.0682) centre (18.4516, -49.9719) ccw
  arc A448 (4.2488, -54.9715) -> (5.0193, -54.9065) centre (0, 0) ccw
  circle A449 centre (0, 0) radius 63.124 construction
  dimension "d31" = 135
  constraints: 896 point on circle, 450 centre point, 1348 other
  measures "d31" diameter of A0
extrude "押し出し1" add sketch "スケッチ1" along normal mid plane 13
sketch "スケッチ5" plane through (0, 0, -6.5) normal (0, 0, -1) x (-1, 0, 0)
  circle A0 centre (0, 0) radius 55.1354 projected
  circle A1 centre (0, 0) radius 67.5 projected
extrude "押し出し3" add sketch "スケッチ5" along normal blind 1
sketch "スケッチ2" plane through (0, 0, 6.5) normal (0, 0, 1) x (1, 0, 0)
  circle A0 centre (0, 0) radius 62.5
  point P0 (-16.1762, 60.3704)
  point P1 (-44.1942, 44.1942)
  point P2 (-60.3704, 16.1762)
  point P3 (-60.3704, -16.1762)
  point P4 (-44.1942, -44.1942)
  point P5 (-16.1762, -60.3704)
  point P6 (16.1762, -60.3704)
  point P7 (44.1942, -44.1942)
  point P8 (60.3704, -16.1762)
  point P9 (60.3704, 16.1762)
  point P10 (44.1942, 44.1942)
  point P11 (16.1762, 60.3704)
  dimension "d3" = 125
  dimension "d6" = 360
  dimension "d21" = 0
  constraints: 1 coincident, 16 other
  measures "d21" vertical distance of point (16.176, 60.37) point (-16.176, 60.37)
hole "穴1" at (-16.1762, 60.3704, 6.5) at (-44.1942, 44.1942, 6.5) at (-60.3704, 16.1762, 6.5) at (-60.3704, -16.1762, 6.5) at (-44.1942, -44.1942, 6.5) at (-16.1762, -60.3704, 6.5) at (16.1762, -60.3704, 6.5) at (44.1942, -44.1942, 6.5) at (60.3704, -16.1762, 6.5) at (60.3704, 16.1762, 6.5) at (44.1942, 44.1942, 6.5) at (16.1762, 60.3704, 6.5) direction (0, 0, -1) diameter 4.3 end through all clearance for "Flat Head Machine Screw" size "M4" standard "Ansi Metric M Profile"
sketch "スケッチ3" plane through (0, 0, 6.5) normal (0, 0, 1) x (1, 0, 0)
  circle A0 centre (-16.1762, 60.3704) radius 2.15 projected
  circle A1 centre (-44.1942, 44.1942) radius 2.15 projected
  circle A2 centre (0, 0) radius 67.5 projected
  circle A3 centre (-44.1942, 44.1942) radius 5
  circle A4 centre (-16.1762, 60.3704) radius 5
  circle A5 centre (0, 0) radius 62.5
  point P0 (-40.52, 47.5855)
  point P1 (-20.9502, 58.8841)
  point P2 (-17.4703, 65.2)
  point P3 (-47.7297, 47.7297)
  constraints: 2 centre point, 2 tangent, 3 other
